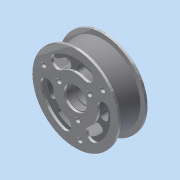
# Autodesk Inventor part: pneumaticwheel_hub
Saved by Autodesk Inventor 2015 (Build 190159000, 159)
## iProperties
Created: 2015-04-12
Part Number: pneumaticwheel_hub
Material: Generic
Document SubType Name: Modeling
Designer: brent
Density: 1 g/cm^3
Appearance: Default
Author: brent
Autodesk Inventor part; units mm, degrees
ref_plane "YZ Plane" through (0, 0, 0) normal (1, 0, 0) x (0, 1, 0)
ref_plane "XZ Plane" through (0, 0, 0) normal (0, 1, 0) x (-1, 0, 0)
ref_plane "XY Plane" through (0, 0, 0) normal (0, 0, 1) x (1, 0, 0)
sketch "Sketch1" plane through (0, 0, 0) normal (1, 0, 0) x (0, 1, 0)
  line L0 (0, 0) -> (-38.1, 0)
  line L1 (-38.1, 0) -> (-38.1, -24.4475)
  line L2 (-38.1, -24.4475) -> (0, -24.4475)
  line L3 (0, -24.4475) -> (0, 0)
  line L4 (0, 0) -> (-11, 0)
  line L5 (-11, 0) -> (-11, -7)
  line L6 (-11, -7) -> (0, -7)
  line L7 (0, -7) -> (0, 0)
  line L8 (0, -7) -> (-10, -7)
  line L9 (-10, -7) -> (-10, -17)
  line L10 (-10, -17) -> (0, -17)
  line L11 (0, -17) -> (0, -7)
  line L12 (0, -17) -> (-11, -17)
  line L13 (-11, -17) -> (-11, -24)
  line L14 (-11, -24) -> (0, -24)
  line L15 (0, -24) -> (0, -17)
  line L16 (0, -24) -> (-11.5, -24)
  line L17 (-11.5, -24) -> (-11.5, -24.4475)
  line L18 (-11.5, -24.4475) -> (0, -24.4475)
  line L19 (0, -24.4475) -> (0, -24)
  arc A0 (-38.1, -24.4475) -> (-38.1, 0) centre (-100.412358, -12.22375) ccw
  line L20 (-30.48, 0) -> (-22.225, 0)
  line L21 (-22.225, 0) -> (-22.225, -24.4475)
  line L22 (-22.225, -24.4475) -> (-30.48, -24.4475)
  line L23 (-30.48, -24.4475) -> (-30.48, 0)
  line L24 (-11, -24) -> (-11.5, -24.4475)
  dimension "d0" = 38.1
  dimension "d1" = 24.4475
  dimension "d2" = 11
  dimension "d3" = 7
  dimension "d4" = 10
  dimension "d5" = 10
  dimension "d6" = 11
  dimension "d7" = 7
  dimension "d8" = 11.5
  dimension "d13" = 63.5
  dimension "d14" = 22.225
  dimension "d15" = 7.62
  constraints: 50 end point, 12 parallel, 6 horizontal, 6 perpendicular, 3 point on line, 2 point on circle, 1 centre point
  measures "d0" distance of L2.end L1.end
  measures "d1" distance of L1.end L0.end
  measures "d2" distance of L6.end L5.end
  measures "d3" distance of L5.end L4.end
  measures "d4" distance of L10.end L9.end
  measures "d5" distance of L9.end L8.end
  measures "d6" distance of L14.end L13.end
  measures "d7" distance of L13.end L12.end
  measures "d8" distance of L18.end L17.end
  measures "d13" radius of A0
  measures "d14" distance between parallel lines of L3 L21
  measures "d15" distance between parallel lines of L1 L23
revolve "Revolution3" add sketch "Sketch1" angle 360 about axis through (0, 0, -24.4475) along (0, 0, 1) contours L5 L6 L9 L12 L13 L16 L17 L2 L21 L0 | L23 L2 A0 L0 | L17 L16 L24
sketch "Sketch5" plane through (0, 0, -24.4475) normal (0, 0, -1) x (-1, 0, 0)
  circle A0 centre (0, 0) radius 22.225
  circle A1 centre (0, 0) radius 30.48
  line L0 (0, 0) -> (0, 22.225)
  line L1 (0, 22.225) -> (0, 30.48)
  line L2 (5.752253, 21.467701) -> (7.888804, 29.441419)
  dimension "d41" = 15
  constraints: 6 end point, 4 point on circle, 2 vertical, 1 point on line
  measures "d41" angle of L1 L2
extrude "Extrusion3" add sketch "Sketch5" against normal up to surface (24.4475 mm away) contours A0 L1 A1 L2 picked at (0.885502, 27.689671)
fillet "Fillet3" radius 3.175 4 edges at (-5.7523, 21.4677, -12.2238) (0, 22.225, -12.2238) (-7.8888, 29.4414, -12.2238) (0, 30.48, -12.2238)
pattern_circular "Circular Pattern3" count 3 over 360 about axis through (0, 0, -12) along (0, 0, 1) of "Extrusion3"
pattern_circular "Circular Pattern5" count 3 over 360 about axis through (0, 0, -12) along (0, 0, 1) of "Fillet3"
sketch "Sketch6" plane through (0, 0, 0) normal (0, 0, 1) x (1, 0, 0)
  circle A0 centre (2.305837, -17.514567) radius 2.4892
  arc A1 (30.159009, -4.411871) -> (3.544186, 30.273241) centre (0, 0) ccw
  arc A2 (-8.3906, 20.580293) -> (-20.485515, -8.619415) centre (0, 0) ccw
  arc A3 (-18.900296, -23.912532) -> (24.445303, -18.205976) centre (0, 0) ccw
  arc A4 (-13.627757, -17.556619) -> (17.70739, -13.431269) centre (0, 0) ccw
  circle A5 centre (0, 0) radius 38.1
  circle A6 centre (0, 0) radius 11
  line L0 (0, 0) -> (3.978438, -30.219239)
  arc A7 (30.159009, -4.411871) -> (3.544186, 30.273241) centre (0, 0) ccw
  circle A8 centre (4.475743, -33.996644) radius 2.4892
  arc A9 (-7.019115, 26.195695) -> (-11.258712, 28.324403) centre (-10.08593, 25.373944) ccw
  arc A10 (0, 25.200781) -> (2.778125, 22.050684) centre (3.175, 25.200781) ccw
  arc A11 (-19.176579, -19.176579) -> (-18.900296, -23.912532) centre (-16.931515, -21.421643) ccw
  arc A12 (21.824517, -12.600391) -> (17.70739, -13.431269) centre (20.237017, -15.350021) ccw
  arc A13 (-11.258712, 28.324403) -> (-27.989489, -12.067266) centre (0, 0) ccw
  arc A14 (-21.824517, -12.600391) -> (-20.485515, -8.619415) centre (-23.412017, -9.85076) ccw
  arc A15 (22.018356, -3.023674) -> (2.778125, 22.050684) centre (0, 0) ccw
  arc A16 (26.195695, -7.019115) -> (30.159009, -4.411871) centre (27.017445, -3.952301) ccw
  line L1 (-17.819643, -17.819643) -> (-19.176579, -19.176579)
  arc A17 (-13.627757, -17.556619) -> (-17.819643, -17.819643) centre (-15.574579, -20.064707) ccw
  line L2 (23.486417, -13.559889) -> (21.824517, -12.600391)
  arc A18 (24.445303, -18.205976) -> (23.486417, -13.559889) centre (21.898917, -16.30952) ccw
  line L3 (-6.522442, 24.342085) -> (-7.019115, 26.195695)
  arc A19 (-8.3906, 20.580293) -> (-6.522442, 24.342085) centre (-9.589257, 23.520335) ccw
  line L4 (-23.486417, -13.559889) -> (-21.824517, -12.600391)
  arc A20 (-27.989489, -12.067266) -> (-23.486417, -13.559889) centre (-25.073917, -10.810259) ccw
  line L5 (0, 27.119779) -> (0, 25.200781)
  arc A21 (3.544186, 30.273241) -> (0, 27.119779) centre (3.175, 27.119779) ccw
  line L6 (24.342085, -6.522442) -> (26.195695, -7.019115)
  arc A22 (22.018356, -3.023674) -> (24.342085, -6.522442) centre (25.163836, -3.455628) ccw
  point P0 (28.309315, -3.887581)
  dimension "d47" = 4.9784
  dimension "d48" = 17.6657
  dimension "d49" = 4.9784
  dimension "d50" = 34.29
  constraints: 2 centre point, 2 end point, 2 point on line, 1 coincident, 1 point on circle, 2 other
  measures "d47" diameter of A0
  measures "d48" distance of point (0, 0) A0.centre
  measures "d49" diameter of A8
  measures "d50" distance of point (0, 0) A8.centre
extrude "Extrusion4" cut sketch "Sketch6" against normal through all contours A0 L0 | L0 A0 | A8
pattern_circular "Circular Pattern4" count 3 over 360 about axis through (0, 0, -12) along (0, 0, 1) of "Extrusion4"
sketch "Sketch12" plane through (0, 0, 0) normal (0, 0, 1) x (1, 0, 0)
  circle A0 centre (-16.320979, 6.760371) radius 2.4892
  circle A1 centre (-31.679829, 13.122215) radius 2.4892
  circle A2 centre (14.015142, 10.754197) radius 2.4892
  circle A3 centre (27.204086, 20.874429) radius 2.4892
  circle A4 centre (2.305837, -17.514567) radius 2.4892
  circle A5 centre (4.475743, -33.996644) radius 2.4892
  arc A6 (-18.900296, -23.912532) -> (24.445303, -18.205976) centre (0, 0) ccw
  arc A7 (-19.176579, -19.176579) -> (-18.900296, -23.912532) centre (-16.931515, -21.421643) ccw
  line L0 (-17.819643, -17.819643) -> (-19.176579, -19.176579)
  arc A8 (-13.627757, -17.556619) -> (-17.819643, -17.819643) centre (-15.574579, -20.064707) ccw
  arc A9 (-13.627757, -17.556619) -> (17.70739, -13.431269) centre (0, 0) ccw
  arc A10 (21.824517, -12.600391) -> (17.70739, -13.431269) centre (20.237017, -15.350021) ccw
  line L1 (23.486417, -13.559889) -> (21.824517, -12.600391)
  arc A11 (24.445303, -18.205976) -> (23.486417, -13.559889) centre (21.898917, -16.30952) ccw
  arc A12 (-11.258712, 28.324403) -> (-27.989489, -12.067266) centre (0, 0) ccw
  arc A13 (-7.019115, 26.195695) -> (-11.258712, 28.324403) centre (-10.08593, 25.373944) ccw
  line L2 (-6.522442, 24.342085) -> (-7.019115, 26.195695)
  arc A14 (-8.3906, 20.580293) -> (-6.522442, 24.342085) centre (-9.589257, 23.520335) ccw
  arc A15 (-8.3906, 20.580293) -> (-20.485515, -8.619415) centre (0, 0) ccw
  arc A16 (-21.824517, -12.600391) -> (-20.485515, -8.619415) centre (-23.412017, -9.85076) ccw
  line L3 (-23.486417, -13.559889) -> (-21.824517, -12.600391)
  arc A17 (-27.989489, -12.067266) -> (-23.486417, -13.559889) centre (-25.073917, -10.810259) ccw
  circle A18 centre (0, 0) radius 38.1
  circle A19 centre (0, 0) radius 11
  arc A20 (22.018356, -3.023674) -> (2.778125, 22.050684) centre (0, 0) ccw
  arc A21 (0, 25.200781) -> (2.778125, 22.050684) centre (3.175, 25.200781) ccw
  line L4 (0, 27.119779) -> (0, 25.200781)
  arc A22 (3.544186, 30.273241) -> (0, 27.119779) centre (3.175, 27.119779) ccw
  arc A23 (30.159009, -4.411871) -> (3.544186, 30.273241) centre (0, 0) ccw
  arc A24 (26.195695, -7.019115) -> (30.159009, -4.411871) centre (27.017445, -3.952301) ccw
  line L5 (24.342085, -6.522442) -> (26.195695, -7.019115)
  arc A25 (22.018356, -3.023674) -> (24.342085, -6.522442) centre (25.163836, -3.455628) ccw
  arc A26 (-11.258712, 28.324403) -> (-27.989489, -12.067266) centre (0, 0) ccw
  line L6 (-22.153961, 20.934001) -> (-27.692452, 26.167501)
  line L7 (-26.958858, 14.221476) -> (-33.698572, 17.776845)
  dimension "d88" = 8.255
  dimension "d111" = 3.175
  constraints: 6 point on circle, 4 end point, 2 point on line
  measures "d88" distance of L6.start L7.start
  measures "d111" distance from line of A1.centre L7
extrude "Extrusion10" cut sketch "Sketch12" against normal blind 15.875 contours A12 L7 A18 L6
fillet "Fillet8" radius 6.35 1 edges at (-22.154, 20.934, -7.9375)
fillet "Fillet9" radius 4.1275 3 edges at (-26.637, 25.1702, -15.875) (-22.3774, 23.1927, -15.875) (-29.85, 15.7466, -15.875)
sketch "Sketch13" plane through (-10.08593, 25.373944, 0) normal (0, 0, 1) x (0.8936747, -0.4487154, 0)
  arc A0 (-14.346023, -7.715091) -> (-6.84385, -4.481195) centre (-12.51949, -1.633457) ccw
  arc A1 (-2.372002, 2.110505) -> (-6.84385, -4.481195) centre (20.399221, -18.15034) ccw
  arc A2 (2.372002, 2.110505) -> (-2.372002, 2.110505) centre (0, 0) ccw
  line L0 (3.64761, 0.676846) -> (2.372002, 2.110505)
  arc A3 (3.666059, -3.523244) -> (3.64761, 0.676846) centre (1.275607, -1.433659) ccw
  arc A4 (3.666059, -3.523244) -> (5.959499, -35.045459) centre (20.399221, -18.15034) ccw
  arc A5 (6.549192, -39.203987) -> (5.959499, -35.045459) centre (3.896682, -37.459048) ccw
  line L1 (5.494535, -40.807187) -> (6.549192, -39.203987)
  arc A6 (0.800491, -41.493865) -> (5.494535, -40.807187) centre (2.842025, -39.062248) ccw
  arc A7 (-10.074624, -17.537822) -> (0.800491, -41.493865) centre (20.399221, -18.15034) ccw
  line L2 (-10.074624, -17.537822) -> (-17.693086, -17.384693)
  arc A8 (-17.693086, -17.384693) -> (-16.090584, -7.191136) centre (20.399221, -18.15034) ccw
  line L3 (-16.090584, -7.191136) -> (-14.346023, -7.715091)
  arc A9 (41.433238, -10.972544) -> (12.987479, 2.802386) centre (20.399221, -18.15034) ccw
  arc A10 (9.091241, 4.370961) -> (12.987479, 2.802386) centre (11.928658, 5.795632) ccw
  line L4 (8.230157, 6.08592) -> (9.091241, 4.370961)
  arc A11 (9.982499, 10.494421) -> (8.230157, 6.08592) centre (11.067574, 7.510592) ccw
  arc A12 (49.331238, -8.560304) -> (9.982499, 10.494421) centre (20.399221, -18.15034) ccw
  arc A13 (46.959235, -12.668733) -> (49.331238, -8.560304) centre (46.317486, -9.559266) ccw
  line L5 (45.079847, -13.056612) -> (46.959235, -12.668733)
  arc A14 (41.433238, -10.972544) -> (45.079847, -13.056612) centre (44.438097, -9.947145) ccw
  circle A15 centre (20.399221, -18.15034) radius 11
  arc A16 (14.238426, -48.001219) -> (50.414672, -23.451575) centre (20.399221, -18.15034) ccw
  arc A17 (11.866424, -43.89279) -> (14.238426, -48.001219) centre (14.880176, -44.891753) ccw
  line L6 (12.470205, -42.071253) -> (11.866424, -43.89279)
  arc A18 (16.098365, -39.95523) -> (12.470205, -42.071253) centre (15.483957, -43.070215) ccw
  arc A19 (16.098365, -39.95523) -> (42.250684, -22.207945) centre (20.399221, -18.15034) ccw
  arc A20 (45.557229, -19.617992) -> (42.250684, -22.207945) centre (45.372322, -22.787603) ccw
  line L7 (47.472969, -19.729752) -> (45.557229, -19.617992)
  arc A21 (50.414672, -23.451575) -> (47.472969, -19.729752) centre (47.288062, -22.899363) ccw
  circle A22 centre (39.653898, -46.523945) radius 2.4892
  circle A23 centre (30.318945, -32.768001) radius 2.4892
  circle A24 centre (35.344145, 12.711503) radius 2.4892
  circle A25 centre (28.098624, -2.250775) radius 2.4892
  circle A26 centre (-13.800381, -20.638576) radius 2.4892
  circle A27 centre (2.780092, -19.432242) radius 2.4892
  line L8 (-17.693086, -17.384693) -> (-10.074624, -17.537822)
  arc A28 (3.666059, -3.523244) -> (5.959499, -35.045459) centre (20.399221, -18.15034) ccw
  line L9 (-1.561268, -21.569049) -> (-9.718021, -22.838855)
  arc A29 (-17.693086, -17.384693) -> (-16.090584, -7.191136) centre (20.399221, -18.15034) ccw
  line L10 (-10.074624, -17.537822) -> (-1.821291, -17.703712)
  dimension "d93" = 10
  constraints: 6 end point, 6 point on circle, 2 point on line
  measures "d93" angle of L8 L9
extrude "Extrusion11" add sketch "Sketch13" against normal up to surface (24.4475 mm away) contours L10 A4 L9 A7
fillet "Fillet10" radius 3.175 3 edges at (-29.0188, 9.3241, -12.2238) (-21.1596, 6.7988, -12.2238) (-19.6575, 10.3698, -12.2238)
fillet "Fillet11" radius 4.1275 1 edges at (-26.9589, 14.2215, -18.0975)
ref_plane "Work Plane3" through (-10.08593, 25.373944, -12.22375) normal (0, 0, 1) x (0.8936747, -0.4487154, 0)
sketch "Sketch14" plane through (-10.08593, 25.373944, 0) normal (0, 0, 1) x (0.8936747, -0.4487154, 0)
  circle A0 centre (-13.800381, -20.638576) radius 2.4892
  circle A1 centre (39.653898, -46.523945) radius 2.4892
  circle A2 centre (35.344145, 12.711503) radius 2.4892
  circle A3 centre (28.098624, -2.250775) radius 2.4892
  circle A4 centre (30.318945, -32.768001) radius 2.4892
  circle A5 centre (2.780092, -19.432242) radius 2.4892
  circle A6 centre (20.399221, -18.15034) radius 42.8625
  circle A7 centre (20.399221, -18.15034) radius 11.5
  dimension "d98" = 85.725
  dimension "d99" = 23
  constraints: 2 centre point, 2 coincident
  measures "d98" diameter of A6
  measures "d99" diameter of A7
extrude "Extrusion12" add sketch "Sketch14" along normal blind 2.38125 separate body
sketch "Sketch15" plane through (0, 0, 2.38125) normal (0, 0, 1) x (1, 0, 0)
  circle A0 centre (0, 0) radius 11.5
  circle A1 centre (-16.320979, 6.760371) radius 2.4892
  circle A2 centre (2.305837, -17.514567) radius 2.4892
  circle A3 centre (14.015142, 10.754197) radius 2.4892
  circle A4 centre (27.204086, 20.874429) radius 2.4892
  circle A5 centre (4.475743, -33.996644) radius 2.4892
  circle A6 centre (-31.679829, 13.122215) radius 2.4892
  circle A7 centre (0, 0) radius 42.8625
  arc A8 (-28.391316, -3.234782) -> (-10.472773, -26.586682) centre (0, 0) ccw construction
  arc A9 (-34.700497, -3.953622) -> (-12.800055, -32.494834) centre (0, 0) ccw
  arc A10 (-22.082134, -2.515941) -> (-8.14549, -20.67853) centre (0, 0) ccw
  arc A11 (-22.082134, -2.515941) -> (-34.700497, -3.953622) centre (-28.391316, -3.234782) ccw
  arc A12 (-12.800055, -32.494834) -> (-8.14549, -20.67853) centre (-10.472773, -26.586682) ccw
  line L0 (0, 0) -> (-28.391316, -3.234782) construction
  line L1 (0, 0) -> (-10.472773, -26.586682) construction
  arc A13 (-8.3906, 20.580293) -> (-18.207093, 12.745681) centre (0, 0) ccw
  line L2 (-16.320979, 6.760371) -> (0, 0) construction
  line L3 (0, 0) -> (-17.632278, -13.529723) construction
  point P0 (0, 0)
  dimension "d102" = 28.575
  dimension "d103" = 62
  dimension "d104" = 12.7
  dimension "d105" = 60
  constraints: 11 point on circle, 8 end point, 5 centre point, 4 tangent, 1 coincident
  measures "d102" radius of A8
  measures "d103" angle of L0 L1
  measures "d104" diameter of A11
  measures "d105" angle of L2 L3
extrude "Extrusion13" cut sketch "Sketch15" against normal blind 2.38125 contours A11 A10 A12 A9 bodies 2
pattern_circular "Circular Pattern7" count 3 over 360 about axis through (0, 0, 0) along (0, 0, 1) of "Extrusion13" bodies 2
mirror "Mirror2" about plane through (-10.08593, 25.373944, -12.22375) normal (0, 0, 1) bodies 2
body "Solid2"
body "Solid3"
body "Solid6"
